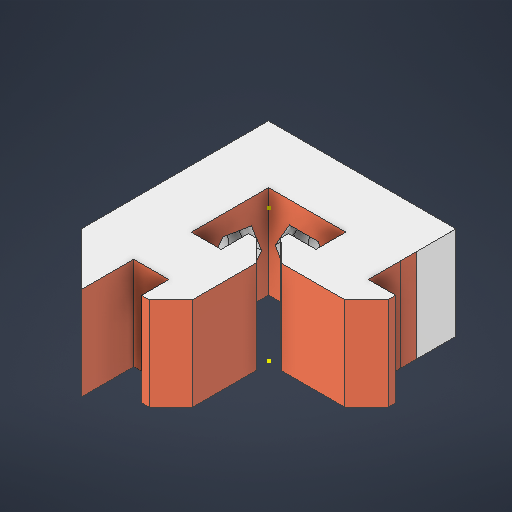
# Autodesk Inventor part: motor_mount_fittest
Saved by Autodesk Inventor 2026.2 (Build 302298010, 298A)
## iProperties
Created: 2026-02-11
Part Number: motor_mount_fittest
Material: ABS Plastic
Document SubType Name: Modeling
Designer: Luke
Density: 1.06 g/cm^3
Appearance: Smooth - White
Author: Luke
Autodesk Inventor part; units mm, degrees
ref_plane "Work Plane1" through (0, 133.5, 0) normal (0, 1, 0) x (1, 0, 0)
sketch "Sketch2" plane through (0, 133.5, 0) normal (0, 1, 0) x (1, 0, 0)
  line L0 (-4.7607, 0) -> (-4.7607, 3.4172)
  line L1 (-4.7607, 3.4172) -> (-7.0894, 5.7459)
  line L2 (-7.0894, 5.7459) -> (-7.9066, 5.7459)
  line L3 (-7.9066, 5.7459) -> (-7.9066, 2.8066)
  line L4 (0, 0) -> (-13.0213, 0) construction
  line L5 (-7.4066, 2.3066) -> (-7.4066, 5.2459)
  line L6 (-7.4066, 5.2459) -> (-7.2965, 5.2459)
  line L7 (-7.2965, 5.2459) -> (-5.2607, 3.2101)
  line L8 (-5.2607, 3.2101) -> (-5.2607, 0.2101)
  line L9 (-3.7133, 3.0016) -> (-3.0065, 3.7094) projected
  line L10 (0, 0) -> (0, 8.149) construction
  line L11 (-11.6066, 2.3066) -> (-17.3293, 2.3066)
  line L12 (-17.3293, 2.3066) -> (-17.3293, 17.3066)
  line L13 (-4.5607, 3.5) -> (-4.5607, -3.5) projected
  line L14 (-7.0066, 5.9459) -> (-4.5607, 3.5) projected
  line L15 (-8.5066, 5.9459) -> (-7.0066, 5.9459) projected
  line L16 (-8.5066, 3.0066) -> (-8.5066, 5.9459) projected
  line L17 (-10.6066, 2.8066) -> (-10.6066, 10.5927)
  line L18 (-11.6066, 2.3066) -> (-11.6066, 0)
  line L19 (-7.9066, 2.8066) -> (-10.6066, 2.8066)
  line L20 (-10.0066, 3.0066) -> (-8.5066, 3.0066) projected
  line L21 (-7.4066, 2.3066) -> (-11.1066, 2.3066)
  line L22 (-11.1066, 0) -> (-11.1066, 2.3066)
  line L23 (-5.2607, 0.2101) -> (-5.2607, 0)
  line L24 (-10.0066, 8.5066) -> (-10.0066, 3.0066) projected
  line L25 (-10.6066, 2.8066) -> (-11.1066, 2.8066) construction
  line L26 (0, 0) -> (-18.7935, 18.7689) construction
  line L27 (-11.6066, 0) -> (-11.6066, 2.3066)
  line L28 (-11.6066, 2.8066) -> (-11.6066, 2.3066)
  line L29 (-11.6066, 2.8066) -> (-10.6066, 2.8066)
  line L30 (-5.2607, 0) -> (-5.2607, 3.2101)
  line L31 (-7.2965, 5.2459) -> (-7.4066, 5.2459)
  line L32 (-7.4066, 2.3066) -> (-7.4066, 5.2459)
  line L33 (-7.4066, 2.3066) -> (-11.1066, 2.3066)
  line L34 (-11.1066, 0) -> (-11.1066, 2.3066)
  line L35 (-12.1161, 0) -> (-4.7607, 0)
  line L36 (-4.7607, 0) -> (-4.7607, -3.4172)
  line L37 (-4.7607, -3.4172) -> (-7.0894, -5.7459)
  line L38 (-7.0894, -5.7459) -> (-7.9066, -5.7459)
  line L39 (-7.9066, -5.7459) -> (-7.9066, -2.8066)
  line L40 (-7.4066, -2.3066) -> (-7.4066, -5.2459)
  line L41 (-7.4066, -5.2459) -> (-7.2965, -5.2459)
  line L42 (-7.2965, -5.2459) -> (-5.2607, -3.2101)
  line L43 (-5.2607, -3.2101) -> (-5.2607, -0.2101)
  line L44 (-7.0066, -5.9459) -> (-4.5607, -3.5)
  line L45 (-8.5066, -5.9459) -> (-7.0066, -5.9459)
  line L46 (-8.5066, -3.0066) -> (-8.5066, -5.9459)
  line L47 (-11.6066, -2.3066) -> (-11.6066, 0)
  line L48 (-7.9066, -2.8066) -> (-10.6066, -2.8066)
  line L49 (-10.0066, -3.0066) -> (-8.5066, -3.0066)
  line L50 (-7.4066, -2.3066) -> (-11.1066, -2.3066)
  line L51 (-11.1066, 0) -> (-11.1066, -2.3066)
  line L52 (-5.2607, -0.2101) -> (-5.2607, 0)
  line L53 (-10.6066, -2.8066) -> (-11.1066, -2.8066) construction
  line L54 (-11.6066, 0) -> (-11.6066, -2.3066)
  line L55 (-11.6066, -2.8066) -> (-11.6066, -2.3066)
  line L56 (-11.6066, -2.8066) -> (-10.6066, -2.8066)
  line L57 (-5.2607, 0) -> (-5.2607, -3.2101)
  line L58 (-7.2965, -5.2459) -> (-7.4066, -5.2459)
  line L59 (-7.4066, -2.3066) -> (-7.4066, -5.2459)
  line L60 (-7.4066, -2.3066) -> (-11.1066, -2.3066)
  line L61 (-11.1066, 0) -> (-11.1066, -2.3066)
  line L62 (-0.0062, 4.7607) -> (-3.4234, 4.7562)
  line L63 (-3.4234, 4.7562) -> (-5.7552, 7.0819)
  line L64 (-5.7552, 7.0819) -> (-5.7563, 7.899)
  line L65 (-5.7563, 7.899) -> (-2.8169, 7.9029)
  line L66 (-2.3163, 7.4035) -> (-5.2556, 7.3997)
  line L67 (-5.2556, 7.3997) -> (-5.2555, 7.2896)
  line L68 (-5.2555, 7.2896) -> (-3.2169, 5.2564)
  line L69 (-3.2169, 5.2564) -> (-0.217, 5.2604)
  line L70 (-3.0065, 3.7094) -> (-3.7133, 3.0016)
  line L71 (-2.3218, 11.6035) -> (-2.3293, 17.3262)
  line L72 (-2.3293, 17.3262) -> (-17.3293, 17.3066)
  line L73 (-5.9551, 6.9988) -> (-3.506, 4.5561)
  line L74 (-5.9571, 8.4988) -> (-5.9551, 6.9988)
  line L75 (-3.0177, 8.5026) -> (-5.9571, 8.4988)
  line L76 (-2.8205, 10.6029) -> (-10.6066, 10.5927)
  line L77 (-2.3218, 11.6035) -> (-0.0152, 11.6065)
  line L78 (-2.8169, 7.9029) -> (-2.8205, 10.6029)
  line L79 (-3.0197, 10.0026) -> (-3.0177, 8.5026)
  line L80 (-2.3163, 7.4035) -> (-2.3211, 11.1035)
  line L81 (-0.0146, 11.1066) -> (-2.3211, 11.1035)
  line L82 (-0.217, 5.2604) -> (-0.0069, 5.2607)
  line L83 (-8.5197, 9.9954) -> (-3.0197, 10.0026)
  line L84 (-2.8205, 10.6029) -> (-2.8211, 11.1029) construction
  line L85 (-0.0152, 11.6065) -> (-2.3218, 11.6035)
  line L86 (-2.8218, 11.6029) -> (-2.3218, 11.6035)
  line L87 (-2.8218, 11.6029) -> (-2.8205, 10.6029)
  line L88 (-0.0069, 5.2607) -> (-3.2169, 5.2564)
  line L89 (-5.2555, 7.2896) -> (-5.2556, 7.3997)
  line L90 (-2.3163, 7.4035) -> (-5.2556, 7.3997)
  line L91 (-2.3163, 7.4035) -> (-2.3211, 11.1035)
  line L92 (-0.0146, 11.1066) -> (-2.3211, 11.1035)
  line L93 (-0.0159, 12.1161) -> (-0.0062, 4.7607)
  line L94 (0.2031, 5.2609) -> (-0.0069, 5.2607)
  line L95 (5.7366, 7.0969) -> (5.7355, 7.9141)
  line L96 (5.2362, 7.4134) -> (5.2363, 7.3034)
  line L97 (5.7355, 7.9141) -> (2.7962, 7.9102)
  line L98 (2.2968, 7.4096) -> (5.2362, 7.4134)
  line L99 (5.2363, 7.3034) -> (3.2031, 5.2649)
  line L100 (3.4109, 4.7651) -> (5.7366, 7.0969)
  line L101 (-0.0062, 4.7607) -> (3.4109, 4.7651)
  line L102 (2.9934, 10.0105) -> (2.9954, 8.5105)
  line L103 (2.7913, 11.6102) -> (2.7926, 10.6102)
  line L104 (2.7913, 11.6102) -> (2.2913, 11.6096)
  line L105 (2.7962, 7.9102) -> (2.7926, 10.6102)
  line L106 (2.2968, 7.4096) -> (5.2362, 7.4134)
  line L107 (2.2913, 11.6096) -> (-0.0152, 11.6065)
  line L108 (-0.0146, 11.1066) -> (2.292, 11.1096)
  line L109 (-0.0146, 11.1066) -> (2.292, 11.1096)
  line L110 (3.2031, 5.2649) -> (0.2031, 5.2609)
  line L111 (0.2031, 5.2609) -> (-0.0069, 5.2607)
  line L112 (-0.0069, 5.2607) -> (3.2031, 5.2649)
  line L113 (-0.0152, 11.6065) -> (2.2913, 11.6096)
  line L114 (5.2363, 7.3034) -> (5.2362, 7.4134)
  line L115 (5.9367, 7.0144) -> (3.494, 4.5652)
  line L116 (2.2968, 7.4096) -> (2.292, 11.1096)
  line L117 (2.2968, 7.4096) -> (2.292, 11.1096)
  line L118 (2.7926, 10.6102) -> (2.792, 11.1102) construction
  line L119 (-0.217, 5.2604) -> (-0.0069, 5.2607)
  line L120 (-2.8218, 11.6029) -> (-2.8286, 16.8256)
  line L121 (-2.8286, 16.8256) -> (-16.8293, 16.8072)
  line L122 (-16.8293, 16.8072) -> (-16.8293, 2.8066)
  line L123 (-16.8293, 2.8066) -> (-11.6066, 2.8066)
  point P0 (-9.2566, 2.3066)
  point P1 (-9.2566, 2.8066)
  point P2 (-9.2566, -2.3066)
  point P3 (-9.2566, -2.8066)
  point P4 (-0.0171, 13.0213)
  point P5 (-2.3187, 9.2535)
  point P6 (-2.8187, 9.2529)
  point P7 (-0.0214, 8.1489)
  point P8 (2.7944, 9.2602)
  point P9 (2.2944, 9.2596)
  point P10 (-5.2607, -0.2101)
  dimension "d73" = 3
  dimension "d74" = 0.2
  dimension "d75" = 0.5
  dimension "d76" = 0.2
  dimension "d77" = 0.2
  dimension "d78" = 0.6
  dimension "d79" = 0.2
  dimension "d80" = 0.5
  dimension "d81" = 0.5
  dimension "d82" = 15
  dimension "d83" = 0.6
  dimension "d84" = 0.5
  dimension "d86" = 0.5
  constraints: 234 end point, 74 symmetric about line, 11 point on line, 10 perpendicular, 7 collinear, 5 horizontal, 4 vertical, 2 midpoint, 2 parallel, 1 vertical alignment, 6 other
  measures "d73" distance of L7.end L8.end
  measures "d74" distance between parallel lines of L0 L13
  measures "d75" distance between parallel lines of L1 L7
  measures "d76" distance between parallel lines of L14 L1
  measures "d77" distance between parallel lines of L15 L2
  measures "d78" distance between parallel lines of L16 L3
  measures "d79" distance between parallel lines of L20 L19
  measures "d80" distance of point (-9.257, 2.307) point (-9.257, 2.807)
  measures "d81" distance between parallel lines of L22 L18
  measures "d82" distance of L11.end L12.end
  measures "d83" distance between parallel lines of L17 L24
  measures "d84" distance of L17.start L25.end
  measures "d86" distance between parallel lines of L12 L122
extrude "Extrusion2" add sketch "Sketch2" along normal blind 30 contours L35 L23 L8 L7 L6 L5 L21 L22 L18 L28 L29 L19 L3 L2 L1 L0 | L36 L37 L38 L39 L48 L56 L55 L47 L35 L51 L50 L40 L41 L42 L43 L52 | L11 L12 L72 L71 L86 L120 L121 L122 L123 L28 | L87 L86 L77 L93 L81 L80 L66 L67 L68 L69 L82 L62 L63 L64 L65 L78 | L107 L104 L103 L105 L97 L95 L100 L101 L93 L94 L110 L99 L96 L98 L116 L108
sketch "Sketch8" plane through (0, 163.5, 0) normal (0, 1, 0) x (1, 0, 0)
  line L0 (2.7962, 7.9102) -> (2.7913, 11.6102) projected
  line L1 (-11.6066, 2.3066) -> (-11.6066, -2.8066) projected
  line L2 (-17.3293, 17.3066) -> (-17.3293, 2.3066) projected
  line L3 (-11.6066, -2.8066) -> (-17.3293, -2.8066)
  line L4 (-17.3293, -2.8066) -> (-17.3293, 2.3066)
  line L5 (-17.3293, 2.3066) -> (-11.6066, 2.3066)
  line L6 (-11.6066, 2.3066) -> (-11.6066, -2.8066)
  line L7 (-2.3293, 17.3262) -> (2.7916, 17.3262)
  line L8 (2.7916, 17.3262) -> (2.7916, 11.3851)
  line L9 (2.7916, 11.3851) -> (-2.3293, 11.3851)
  line L10 (-2.3293, 11.3851) -> (-2.3293, 17.3262)
  point P0 (0, 0)
  constraints: 16 end point, 4 parallel, 2 horizontal, 2 perpendicular, 1 point on line
extrude "Extrusion5" add sketch "Sketch8" against normal blind 30
sketch "Sketch10" plane through (0, 163.5, 0) normal (0, 1, 0) x (1, 0, 0)
  point P0 (0, 0)
sketch "Sketch11" plane through (0, 163.5, 0) normal (0, 1, 0) x (1, 0, 0)
  line L0 (-2.3211, 11.1035) -> (2.292, 11.1096) projected
  line L1 (-17.118, 17.0457) -> (-2.3422, 17.0457)
  line L2 (-2.3422, 17.0457) -> (-2.3422, 11.1035)
  line L3 (-2.3422, 11.1035) -> (-17.118, 11.1035)
  line L4 (-17.118, 11.1035) -> (-17.118, 17.0457)
  line L5 (-11.1066, 2.3066) -> (-7.4066, 2.3066) projected
  line L6 (-17.118, 17.0457) -> (-11.1066, 17.0457)
  line L7 (-11.1066, 17.0457) -> (-11.1066, 2.3066)
  line L8 (-11.1066, 2.3066) -> (-17.118, 2.3066)
  line L9 (-17.118, 2.3066) -> (-17.118, 17.0457)
  line L10 (-7.9066, -2.8066) -> (-17.3293, -2.8066) projected
  line L11 (-11.6847, -2.8066) -> (-11.6847, -8.4511)
  line L12 (-11.6847, -2.8066) -> (-6.0401, -2.8066) construction
  line L13 (-11.6847, -8.4511) -> (-17.3293, -2.8066)
  line L14 (2.7962, 7.9102) -> (2.7916, 11.3851) projected
  line L15 (2.7918, 11.2643) -> (8.8539, 11.2643)
  line L16 (2.7916, 17.3262) -> (-2.3293, 17.3262) projected
  line L17 (2.7916, 17.3262) -> (8.8539, 11.2643)
  line L18 (2.7947, 9.0187) -> (2.7916, 17.3262)
  point P0 (0, 0)
  point P1 (-11.1066, 11.1035)
  point P2 (2.7939, 11.2643)
  point P3 (2.7913, 11.6102)
  dimension "d147" = 45
  dimension "d149" = 44.999
  constraints: 28 end point, 4 horizontal, 4 parallel, 4 point on line, 3 perpendicular, 1 vertical
  measures "d147" angle of L13 L11
  measures "d149" angle of L15 L17
extrude "Extrusion6" add sketch "Sketch11" against normal up to surface (30 mm away) contours L1 L7 L3 L4 | L1 L2 L3 L7 | L3 L7 L8 L9
extrude "Extrusion7" add sketch "Sketch11" against normal blind 30 contours L11 L13 L10 | L18 L17 L15
extrude "Extrusion8" add sketch "Sketch2" along normal up to surface (30 mm away) contours L35 L22 L21 L5 L6 L7 L8 L23 | L52 L43 L42 L41 L40 L50 L51 L35 | L93 L82 L69 L68 L67 L66 L80 L81 | L108 L116 L98 L96 L99 L110 L94 L93
sketch "Sketch6" plane through (-11.6066, 133.5, -2.3066) normal (-1, 0, 0) x (0, 0, 1)
  line L0 (-15, 30) -> (0, 30) projected
  line L1 (0, 30) -> (5.1131, 30) projected
  line L2 (0, 30) -> (5.1131, 30)
  line L3 (2.5566, 30) -> (2.5566, 0)
  line L4 (0, 0) -> (5.1131, 0) projected
  circle A0 centre (2.5566, 15) radius 2.5
  dimension "d121" = 5
  constraints: 4 end point, 3 midpoint, 1 centre point, 1 coincident, 1 collinear
  measures "d121" diameter of A0
sketch "Sketch7" plane through (-2.3218, 133.5, -11.6035) normal (-0.0013, 0, -1) x (-1, 0, 0.0013)
  line L0 (-5.1131, 0) -> (-5.1131, 30) projected
  line L1 (0, 30) -> (15, 30) projected
  line L2 (-5.1131, 30) -> (0, 30)
  line L3 (-2.5566, 30) -> (-2.5566, 0)
  line L4 (0, 0) -> (-4.6131, 0) projected
  circle A0 centre (-2.5566, 15) radius 2.5
  dimension "d122" = 5
  constraints: 4 end point, 2 midpoint, 1 centre point, 1 coincident, 1 collinear, 1 point on line, 1 vertical
  measures "d122" diameter of A0
ref_plane "Work Plane2" through (0, 148.5, 0) normal (0, 1, 0) x (1, 0, 0)
sketch "Sketch13" plane through (0, 148.5, 0) normal (0, 1, 0) x (1, 0, 0)
  line L0 (14.8441, 67.8647) -> (-12.7331, 95.4419) construction
  line L1 (-12.7331, 95.4419) -> (-32.8856, 75.2893) construction
  line L2 (-32.8856, 75.2893) -> (-5.3085, 47.7122) construction
  line L3 (-5.3085, 47.7122) -> (14.8441, 67.8647) construction
  line L4 (-2.3293, 17.3262) -> (-17.3293, 17.3066) projected
  line L5 (0, 0) -> (-17.3293, 17.3066) construction
  line L6 (-17.3293, 17.3066) -> (-17.3293, 17.3066) construction
  line L7 (-39.3305, 39.3078) -> (-18.1173, 60.521) construction
  line L8 (-17.3293, 17.3066) -> (-17.3293, -2.8066) projected
  line L9 (-17.3293, 17.3066) -> (-42.078, 42.0553) construction
  line L10 (-42.078, 42.0553) -> (-20.8648, 63.2685) construction
  line L11 (20.1474, 71.7538) -> (-3.8943, 47.7122)
  line L12 (-49.1491, 77.4106) -> (-6.7227, 34.9842) construction
  line L13 (-6.7227, 34.9842) -> (-35.0069, 6.7) construction
  line L14 (-35.0069, 6.7) -> (-77.4334, 49.1264) construction
  line L15 (-77.4334, 49.1264) -> (-49.1491, 77.4106) construction
  line L16 (-49.1491, 77.4106) -> (-35.0069, 6.7) construction
  line L17 (-6.7227, 34.9842) -> (-77.4334, 49.1264) construction
  line L18 (-84.5025, 56.1955) -> (-27.9339, -0.3731) construction
  line L19 (-27.9339, -0.3731) -> (-35.005, -7.4441) construction
  line L20 (-35.005, -7.4441) -> (-91.5735, 49.1244) construction
  line L21 (-91.5735, 49.1244) -> (-84.5025, 56.1955) construction
  line L22 (-84.5025, 56.1955) -> (-35.005, -7.4441) construction
  line L23 (-27.9339, -0.3731) -> (-91.5735, 49.1244) construction
  line L24 (-56.2182, 84.4797) -> (0.3504, 27.9112) construction
  line L25 (0.3504, 27.9112) -> (7.4214, 34.9823) construction
  line L26 (7.4214, 34.9823) -> (-49.1471, 91.5508) construction
  line L27 (34.4866, -31.2721) -> (31.3132, -31.2721) construction
  line L28 (-30.5205, 27.2872) -> (-27.9594, 27.2872) construction
  line L29 (-29.24, 26.4576) -> (-29.24, 28.1733) construction
  line L30 (-32.8856, 75.2893) -> (-35.005, 77.4087) construction
  line L31 (-3.8943, 47.7122) -> (25.244, 47.7122) construction
  line L32 (-3.0114, 46.8293) -> (-3.7185, 46.1222) construction
  line L33 (-3.8943, 47.7122) -> (-33.9077, 77.7257) construction
  line L34 (-3.8943, 47.7122) -> (38.5512, 47.7122) construction
  line L35 (-2.3293, 17.3262) -> (2.7916, 17.3262) projected
  line L36 (2.7916, 17.3262) -> (14.6413, 29.1766)
  line L37 (2.7916, 17.3262) -> (8.8539, 11.2643) projected
  line L38 (8.8539, 11.2643) -> (26.7661, 29.1766)
  line L39 (8.8539, 11.2643) -> (34.1856, 11.2643) construction
  line L40 (26.7661, 29.1766) -> (14.6413, 29.1766) construction
  line L41 (26.7661, 29.1766) -> (9.2392, 46.7035)
  line L42 (26.7661, 29.1766) -> (66.5529, 29.1766) construction
  line L43 (9.2392, 46.7035) -> (34.2895, 71.7538)
  line L44 (9.2392, 46.7035) -> (44.6657, 46.7035) construction
  line L45 (10.4159, 62.0223) -> (17.487, 54.9513) construction
  line L46 (10.4159, 62.0223) -> (20.4159, 62.0223) construction
  line L47 (8.8539, 11.2643) -> (2.7916, 17.3262)
  line L48 (-27.1184, 82.4708) -> (-4.1184, 82.4708) construction
  line L49 (15.4451, 17.8556) -> (9.3827, 23.9177) construction
  line L50 (20.1474, 71.7538) -> (3.8839, 88.0172)
  line L51 (20.1474, 71.7538) -> (43.1474, 71.7538) construction
  line L52 (34.2895, 71.7538) -> (10.955, 95.0883)
  line L53 (34.2895, 71.7538) -> (67.2895, 71.7538) construction
  line L54 (10.955, 95.0883) -> (3.8839, 88.0172) construction
  line L55 (-20.8648, 63.2685) -> (3.8839, 88.0172) construction
  line L56 (-12.3795, 104.2807) -> (-36.4212, 80.2391)
  line L57 (-37.4298, 93.3725) -> (-12.3795, 118.4228)
  line L58 (-12.3795, 104.2807) -> (3.8839, 88.0172)
  line L59 (-12.3795, 118.4228) -> (10.955, 95.0883)
  line L60 (-37.4298, 93.3725) -> (-43.4922, 87.3101)
  line L61 (-37.4298, 93.3725) -> (-28.8563, 93.3725) construction
  line L62 (-43.4922, 87.3101) -> (-36.4212, 80.2391)
  line L63 (-7.3926, 51.2105) -> (-8.0997, 50.5034) construction
  line L64 (9.4143, 82.4868) -> (16.4854, 89.5579) construction
  line L65 (-27.8481, 88.8121) -> (-34.9192, 95.8832) construction
  line L66 (-3.8943, 47.7122) -> (14.6413, 29.1766)
  point P0 (-29.3501, 73.168)
  point P1 (-59.7537, 24.3757)
  point P2 (-0.0052, 84.1282)
  dimension "d147" = 45
  dimension "d203" = 45
  dimension "d204" = 4
  dimension "d127" = 28.5
  dimension "d129" = 30
  dimension "d131" = 35
  dimension "d132" = 17
  dimension "d134" = 60
  dimension "d136" = 40
  dimension "d137" = 80
  dimension "d138" = 10
  dimension "d139" = 135
  dimension "d140" = 1
  dimension "d144" = 1
  dimension "d145" = 135
  dimension "d150" = 45
  dimension "d151" = 45
  dimension "d152" = 135
  dimension "d153" = 45
  dimension "d157" = 45
  dimension "d158" = 10
  dimension "d164" = 23
  dimension "d165" = 135
  dimension "d166" = 135
  dimension "d167" = 90
  dimension "d169" = 90
  dimension "d170" = 135
  dimension "d192" = 1
  dimension "d193" = 10
  dimension "d194" = 10
  dimension "d195" = 34
  dimension "d196" = 90
  constraints: 126 end point, 22 point on line, 12 horizontal, 12 perpendicular, 7 equal length, 7 parallel, 7 symmetric about line, 4 midpoint, 2 collinear, 1 coincident, 1 vertical
  measures "d127" distance of L2.end L0.start
  measures "d129" distance of L7.start L7.end
  measures "d131" distance of L9.start L9.end
  measures "d132" distance of L1.end L10.end
  measures "d134" distance of L12.start L12.end
  measures "d136" distance of L12.end L13.end
  measures "d137" distance of L18.start L18.end
  measures "d138" distance of L18.end L19.end
  measures "d139" angle of L29 L6
  measures "d140" distance between parallel lines of L3 L11
  measures "d144" distance of L32.start L32.end
  measures "d145" angle of L34 L33
  measures "d150" angle of L39 L38
  measures "d151" angle of L40 L38
  measures "d152" angle of L42 L41
  measures "d153" angle of L44 L43
  measures "d157" angle of L45 L46
  measures "d158" distance of L45.start L45.end
  measures "d164" distance of L11.start L50.end
  measures "d165" angle of L51 L50
  measures "d166" angle of L53 L52
  measures "d167" angle of L54 L50
  measures "d169" angle of L55 L26
  measures "d170" angle of L60 L61
  measures "d192" distance of L63.start L63.end
  measures "d193" distance of L64.start L64.end
  measures "d194" distance of L65.start L65.end
  measures "d195" distance of L11.start L11.end
  measures "d196" angle of L37 L36
extrude "Extrusion11" add sketch "Sketch13" along normal mid plane 10
ref_plane "Work Plane4" through (0, 148.5, 0) normal (0, 1, 0) x (1, 0, 0)
sketch "Sketch16" plane through (0, 148.5, 0) normal (0, 1, 0) x (1, 0, 0)
  line L0 (20.1474, 71.7538) -> (-3.8943, 47.7122) projected
  line L1 (-3.8943, 47.7122) -> (20.1474, 71.7538)
  line L2 (20.1474, 71.7538) -> (-12.3795, 104.2807)
  line L3 (-12.3795, 104.2807) -> (-36.4212, 80.2391)
  line L4 (-35.658, 86.6591) -> (-12.3795, 109.9375)
  line L5 (-12.3795, 109.9375) -> (25.8042, 71.7538)
  line L6 (25.8042, 71.7538) -> (-1.0658, 44.8837)
  line L7 (-36.4212, 80.2391) -> (-12.3795, 104.2807)
  line L8 (-15.208, 107.1091) -> (-39.2496, 83.0675)
  line L9 (-39.2496, 83.0675) -> (-36.4212, 80.2391)
  line L10 (-1.0658, 44.8837) -> (-3.8943, 47.7122)
  line L11 (-3.8943, 47.7122) -> (14.6413, 29.1766) projected
  line L12 (-43.4922, 87.3101) -> (-36.4212, 80.2391) projected
  point P0 (0, 0)
  point P1 (12.3692, 58.3188)
  dimension "d180" = 4
  dimension "d181" = 4
  dimension "d182" = 46
  dimension "d183" = 4
  constraints: 20 end point, 4 collinear, 3 parallel, 1 midpoint, 1 perpendicular
  measures "d180" distance from line of L0 point (12.369, 58.319)
  measures "d181" distance between parallel lines of L4 L3
  measures "d182" distance of L0.start L2.end
  measures "d183" distance between parallel lines of L5 L2
extrude "Extrusion12" add sketch "Sketch16" against normal blind 19.25
extrude "Extrusion14" add sketch "Sketch16" along normal blind 14.25
sketch "Sketch18" plane through (0, 129.25, 0) normal (0, -1, 0) x (1, 0, 0)
  line L0 (-3.8943, -47.7122) -> (20.1474, -71.7538) projected
  line L1 (20.1474, -71.7538) -> (-3.8943, -47.7122)
  line L2 (-3.8943, -47.7122) -> (-36.4212, -80.2391)
  line L3 (-36.4212, -80.2391) -> (-12.3795, -104.2807)
  line L4 (-12.3795, -104.2807) -> (20.1474, -71.7538)
  point P0 (0, 0)
  constraints: 8 end point, 3 equal length, 1 perpendicular
extrude "Extrusion15" add sketch "Sketch18" against normal blind 5
ref_plane "Work Plane5" through (-231821.5246, 143.5, 231819.1141) normal (0.7071, 0, 0.7071) x (0, 1, 0)
sketch "Sketch19" plane through (-231821.5246, 143.5, 231819.1141) normal (0.7071, 0, 0.7071) x (0, 1, 0)
  line L0 (20, -327857.6653) -> (10, -327857.6653) projected
  line L1 (17.5, -327857.6653) -> (10, -327865.1653)
  line L2 (10, -327874.4237) -> (10, -327857.6653) projected
  line L3 (17.5, -327857.6653) -> (28.1066, -327857.6653) construction
  line L4 (17.5, -327857.6653) -> (10, -327857.6653)
  line L5 (10, -327865.1653) -> (10, -327857.6653)
  dimension "d197" = 135
  dimension "d198" = 2.5
  constraints: 8 end point, 2 collinear, 2 point on line, 1 equal length, 1 horizontal
  measures "d197" angle of L1 L3
  measures "d198" distance of L0.start L1.start
extrude "Extrusion16" add sketch "Sketch19" along normal mid plane 4
mirror "Mirror2" about plane through (0, 148.5, 0) normal (0, 1, 0) of "Extrusion16"
sketch "Sketch20" plane through (0, 148.5, 0) normal (0, 1, 0) x (1, 0, 0)
  line L0 (0, 0) -> (-56.5685, 56.5685) construction
  line L1 (0, 0) -> (80, 0) construction
  dimension "d201" = 80
  dimension "d202" = 135
  constraints: 4 end point, 1 equal length, 1 horizontal
  measures "d201" distance of L0.start L0.end
  measures "d202" angle of L1 L0
sketch "Sketch21" plane through (0, 148.5, 0) normal (0, 1, 0) x (1, 0, 0)
  point P0 (0, 0)
sketch "Sketch22" plane through (0, 148.5, 0) normal (0, 1, 0) x (1, 0, 0)
  line L0 (23.9377, 32.005) -> (23.9377, 61.4019)
  line L1 (34.2895, 71.7538) -> (9.2392, 46.7035) projected
  line L2 (9.2392, 46.7035) -> (26.7661, 29.1766) projected
  line L3 (-1.0658, 44.8837) -> (14.6413, 29.1766) projected
  line L4 (7.6413, 36.1766) -> (7.6413, 22.1762)
  line L5 (14.6413, 29.1766) -> (2.7916, 17.3262) projected
  point P0 (0, 0)
  dimension "d203" = 45
  dimension "d204" = 4
  dimension "d207" = 45
  dimension "d208" = 7
  constraints: 4 end point, 4 point on line, 1 coincident
  measures "d203" angle of L0 L2
  measures "d204" distance of L2.end L0.start
  measures "d207" angle of L3 L4
  measures "d208" distance from line of point (14.641, 29.177) L4
extrude "Extrusion17" add sketch "Sketch22" along normal mid plane 4
sketch "Sketch23" plane through (0, 162.75, 0) normal (0, 1, 0) x (1, 0, 0)
  point P0 (0, 0)
sketch "Sketch25" plane through (0, 162.75, 0) normal (0, 1, 0) x (1, 0, 0)
  point P0 (0, 0)
sketch "Sketch26" plane through (0, 162.75, 0) normal (0, 1, 0) x (1, 0, 0)
  line L0 (-12.3795, 104.2807) -> (20.1474, 71.7538) projected
  line L1 (20.1474, 71.7538) -> (-12.3795, 104.2807)
  line L2 (-12.3795, 104.2807) -> (-36.4212, 80.2391)
  line L3 (-36.4212, 80.2391) -> (-3.8943, 47.7122)
  line L4 (-3.8943, 47.7122) -> (20.1474, 71.7538)
  line L5 (-37.1283, 80.2391) -> (-12.3795, 104.9878)
  line L6 (-12.3795, 104.9878) -> (20.8545, 71.7538)
  line L7 (20.8545, 71.7538) -> (-3.8943, 47.005)
  line L8 (-3.8943, 47.005) -> (-37.1283, 80.2391)
  point P0 (0, 0)
  dimension "d210" = 0.5
  constraints: 16 end point, 5 equal length, 2 perpendicular, 3 other
  measures "d210" distance between parallel lines of L2 L5
extrude "Extrusion18" cut sketch "Sketch26" against normal up to surface (28.5 mm away) contours L0 L4 L3 L2 | L5 L6 L7 L8
sketch "Sketch27" plane through (-17.3293, 133.5, -17.3066) normal (-1, 0, 0) x (0, 0, 1)
  line L0 (-0.0197, 20) -> (-0.0197, 10) projected
  line L1 (-0.0197, 15) -> (9.9803, 15) construction
  circle A0 centre (9.9803, 15) radius 1.5
  point P0 (17.3066, -133.5)
  dimension "d213" = 10
  dimension "d214" = 3
  constraints: 2 end point, 1 centre point, 1 coincident, 1 horizontal, 1 midpoint
  measures "d213" distance of L1.start L1.end
  measures "d214" diameter of A0
hole "Hole3" at (-17.3293, 148.5, -7.3262) direction (1, 0, 0) diameter 3 depth 8 tip angle 118 counterbore diameter 5.5 counterbore depth 2.5
sketch "Sketch28" plane through (-17.3293, 133.5, -17.3066) normal (-0.0013, 0, -1) x (-1, 0, 0.0013)
  ellipse E0 centre (0.0131, 15) end of major axis (0.0131, 12.25) minor radius 0.0036 projected
  line L0 (0.0131, 15) -> (-9.9869, 15) construction
  line L1 (0.0264, 30) -> (0.0264, 0) projected
  line L2 (0.0131, 15) -> (0.0264, 30) construction
  circle A0 centre (-9.9869, 15) radius 1.25
  point P0 (-17.3066, -133.5)
  dimension "d222" = 10
  dimension "d223" = 2.5
  constraints: 4 end point, 1 centre point, 1 coincident, 1 horizontal, 1 other
  measures "d222" distance of L0.start L0.end
  measures "d223" diameter of A0
hole "Hole4" at (-7.3424, 148.5, -17.3197) direction (0.0013, 0, 1) diameter 3 depth 8 tip angle 118 counterbore diameter 5.5 counterbore depth 2.5
sketch "Sketch29" plane through (0, 163.5, 0) normal (0, 1, 0) x (1, 0, 0)
  line L0 (-17.3293, 17.3066) -> (-17.3293, -2.8066) projected
  line L1 (-17.3293, 17.3066) -> (46.0524, 17.3262)
  line L2 (46.0524, 17.3262) -> (46.0222, 114.3129)
  line L3 (46.0222, 114.3129) -> (-17.3594, 114.2932)
  line L4 (-17.3594, 114.2932) -> (-17.3293, 17.3066)
  line L5 (-110.0198, 149.1927) -> (107.7957, 149.2603)
  line L6 (107.7957, 149.2603) -> (107.8339, 26.2715)
  line L7 (107.8339, 26.2715) -> (-109.9816, 26.2039)
  line L8 (-109.9816, 26.2039) -> (-110.0198, 149.1927)
  line L9 (2.7916, 11.3851) -> (2.7916, 17.3262) projected
  line L10 (2.7916, 17.3262) -> (18.2078, 17.3176)
  line L11 (18.2078, 17.3176) -> (18.2026, 7.9013)
  line L12 (18.2026, 7.9013) -> (2.7863, 7.91)
  line L13 (2.7863, 7.91) -> (2.7916, 17.3262)
  point P0 (0, 0)
  constraints: 24 end point, 7 parallel, 3 perpendicular, 1 point on line
extrude "Extrusion19" cut sketch "Sketch29" against normal blind 800 contours L7 L4 L3 L2 | L2 L3 L4 L7 L8 L5 L6
sketch "Sketch30" plane through (0, 163.5, 0) normal (0, 1, 0) x (1, 0, 0)
  line L0 (2.7962, 7.9102) -> (2.7916, 11.3851) projected
  line L1 (2.7932, 10.184) -> (29.194, 10.184)
  line L2 (29.194, 10.184) -> (29.194, 30.9791)
  line L3 (29.194, 30.9791) -> (2.7932, 30.9791)
  line L4 (2.7932, 30.9791) -> (2.7932, 10.184)
  point P0 (0, 0)
  constraints: 8 end point, 2 parallel, 1 horizontal, 1 perpendicular, 1 point on line
extrude "Extrusion20" cut sketch "Sketch30" against normal blind 800
sketch "Sketch31" plane through (0, 163.5, 0) normal (0, 1, 0) x (1, 0, 0)
  line L0 (-21.2517, 19.0362) -> (12.6228, 19.0362)
  line L1 (12.6228, 19.0362) -> (12.6228, -13.439)
  line L2 (12.6228, -13.439) -> (-21.2517, -13.439)
  line L3 (-21.2517, -13.439) -> (-21.2517, 19.0362)
  point P0 (0, 0)
  constraints: 8 end point, 2 parallel, 1 horizontal, 1 perpendicular
extrude "Extrusion21" cut sketch "Sketch31" against normal blind 10
sketch "Sketch32" plane through (0, 133.5, 0) normal (0, -1, 0) x (1, 0, 0)
  line L0 (-28.7146, 16.4708) -> (13.0892, 16.4708)
  line L1 (13.0892, 16.4708) -> (13.0892, -20.5521)
  line L2 (13.0892, -20.5521) -> (-28.7146, -20.5521)
  line L3 (-28.7146, -20.5521) -> (-28.7146, 16.4708)
  point P0 (0, 0)
  constraints: 8 end point, 2 parallel, 1 horizontal, 1 perpendicular
extrude "Extrusion22" cut sketch "Sketch32" against normal blind 10
sketch "Sketch33" plane through (-11.1066, 153.5, -2.8066) normal (1, 0, 0) x (0, 0, -1)
  circle A0 centre (4.5197, -5) radius 1.5 projected
  line L0 (5.6218, -7.8546) -> (2.5986, -7.3817)
  line L1 (2.5986, -7.3817) -> (1.4965, -4.5271)
  line L2 (1.4965, -4.5271) -> (3.4176, -2.1454)
  line L3 (3.4176, -2.1454) -> (6.4408, -2.6183)
  line L4 (6.4408, -2.6183) -> (7.5429, -5.4729)
  line L5 (7.5429, -5.4729) -> (5.6218, -7.8546)
  point P0 (-2.8066, -153.5)
  dimension "d247" = 5.3
  constraints: 12 end point, 1 coincident, 13 other
  measures "d247" distance between parallel lines of L4 L1
extrude "Extrusion23" cut sketch "Sketch33" against normal blind 2 contours A0 | L0 L1 L2 L3 L4 L5
sketch "Sketch34" plane through (-11.1066, 153.5, -11.1035) normal (0, 0, 1) x (1, 0, 0)
  ellipse E0 centre (3.7675, -5) end of major axis (3.7675, -3.5) minor radius 1.5 projected
  line L0 (6.8274, -5) -> (5.2974, -7.65)
  line L1 (5.2974, -7.65) -> (2.2375, -7.65)
  line L2 (2.2375, -7.65) -> (0.7075, -5)
  line L3 (0.7075, -5) -> (2.2375, -2.35)
  line L4 (2.2375, -2.35) -> (5.2974, -2.35)
  line L5 (5.2974, -2.35) -> (6.8274, -5)
  point P0 (11.1066, -153.5)
  dimension "d245" = 5.3
  constraints: 12 end point, 1 coincident, 14 other
  measures "d245" distance between parallel lines of L3 L0
extrude "Extrusion24" cut sketch "Sketch34" against normal blind 2 contours E0 | L0 L1 L2 L3 L4 L5
equation "\"hole_diam\" = 5"
body "Solid1"
